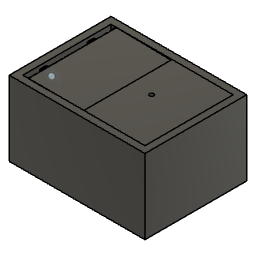
Useless box v2 (Autodesk Fusion 360 design; units mm, degrees)
Autodesk Fusion 360 part; units mm, degrees
sketch "Esquisse1" plane through (0, 0, 0) normal (0, 1, 0) x (1, 0, 0)
  line L0 (0, 0) -> (200, 0)
  line L1 (200, 0) -> (200, -150)
  line L2 (200, -150) -> (0, -150)
  line L3 (0, -150) -> (0, 0)
  line L4 (10, -10) -> (190, -10)
  line L5 (190, -10) -> (190, -140)
  line L6 (190, -140) -> (10, -140)
  line L7 (10, -140) -> (10, -10)
  dimension "d1" = 200
  dimension "d2" = 150
  constraint horizontal L0
  constraint vertical L1
  constraint horizontal L2
  constraint vertical L3
  constraint coincident L0.start L3.end
  constraint horizontal L4
  constraint vertical L5
  constraint horizontal L6
  constraint vertical L7
  measures "d1" distance of L0.start L0.end
  measures "d2" distance of L0 L2
sketch "Esquisse2" plane through (100, 0, 75) normal (0, 1, 0) x (1, 0, 0)
  line L0 (-90, 65) -> (90, 65)
  line L1 (90, 65) -> (90, -65)
  line L2 (90, -65) -> (-90, -65)
  line L3 (-90, -65) -> (-90, 65)
  constraint horizontal L0
  constraint vertical L1
  constraint horizontal L2
  constraint vertical L3
extrude "Extrusion1" add sketch "Esquisse1" along normal blind 20 contours L0 L1 L2 L3 | L4 L5 L6 L7 makes body 1
sketch "Esquisse3" plane through (100, 0, 75) normal (0, 1, 0) x (1, 0, 0)
extrude "Extrusion2" add sketch "Esquisse1" along normal blind 90 from surface at 20 bodies 1
sketch "Esquisse4" plane through (190, 0, 0) normal (-1, 0, 0) x (0, 0, 1)
  line L0 (10, 20) -> (140, 20)
  line L1 (140, 20) -> (140, 110)
  line L2 (140, 110) -> (10, 110)
  line L3 (10, 110) -> (10, 20)
  line L4 (10, 110) -> (140, 110)
  line L5 (140, 110) -> (140, 100)
  line L6 (140, 100) -> (10, 100)
  line L7 (10, 100) -> (10, 110)
  constraint horizontal L4
  constraint vertical L5
  constraint horizontal L6
  constraint vertical L7
  constraint coincident L1 L5.end
  constraint coincident L2.end L3.start
extrude "Extrusion3" add sketch "Esquisse4" along normal blind 90 separate body contours L1 L2 L3 L4 L5 L6 L7 makes body 2
sketch "Esquisse5" plane through (10, 0, 0) normal (1, 0, 0) x (0, 0, -1)
  line L0 (-140, 20) -> (-10, 20)
  line L1 (-10, 20) -> (-10, 110)
  line L2 (-10, 110) -> (-140, 110)
  line L3 (-140, 110) -> (-140, 20)
  line L4 (-115, 105) -> (-105, 105)
  line L5 (-105, 105) -> (-105, 90)
  line L6 (-105, 90) -> (-115, 90)
  line L7 (-115, 90) -> (-115, 105)
  line L8 (-35, 105) -> (-45, 105)
  line L9 (-45, 105) -> (-45, 90)
  line L10 (-45, 90) -> (-35, 90)
  line L11 (-35, 90) -> (-35, 105)
  constraint horizontal L4
  constraint vertical L5
  constraint horizontal L6
  constraint vertical L7
  constraint horizontal L8
  constraint vertical L9
  constraint horizontal L10
  constraint vertical L11
extrude "Extrusion4" add sketch "Esquisse5" along normal blind 20 separate body contours L4 L5 L6 L7 | L8 L9 L10 L11 makes body 3 at (16.6667, 100, 105) makes body 4 at (16.6667, 95, 35)
sketch "Esquisse6" plane through (0, 0, 105) normal (0, 0, -1) x (-1, 0, 0)
  line L0 (-10, 90) -> (-10, 105)
  line L1 (-10, 105) -> (-30, 105)
  line L2 (-30, 105) -> (-30, 90)
  line L3 (-30, 90) -> (-10, 90)
  circle A0 centre (-17.5, 95) radius 2.5
  dimension "d12" = 5
  measures "d12" diameter of A0
extrude "Extrusion5" cut sketch "Esquisse6" along normal blind 70 and the other way blind 10 contours A0 bodies 3 4
sketch "Esquisse7" plane through (0, 110, 0) normal (0, 1, 0) x (-1, 0, 0)
  line L0 (-190, 140) -> (-190, 10)
  line L1 (-190, 10) -> (-100, 10)
  line L2 (-100, 10) -> (-100, 140)
  line L3 (-100, 140) -> (-190, 140)
  circle A0 centre (-130, 70) radius 3
  dimension "d17" = 6
  measures "d17" diameter of A0
extrude "Extrusion6" cut sketch "Esquisse7" against normal blind 10 contours A0 bodies 2
sketch "Esquisse1 (2)" plane through (0, 110, 0) normal (0, 1, 0) x (-1, 0, 0) in component "couvercle"
  line L0 (-190, 140) -> (-10, 140)
  line L1 (-10, 140) -> (-10, 10)
  line L2 (-10, 10) -> (-190, 10)
  line L3 (-190, 10) -> (-190, 140)
  line L4 (0, 150) -> (-200, 150)
  line L5 (-200, 150) -> (-200, 0)
  line L6 (-200, 0) -> (0, 0)
  line L7 (0, 0) -> (0, 150)
  line L8 (-10, 114.9857) -> (-30, 114.9857)
  line L9 (-30, 114.9857) -> (-30, 105)
  line L10 (-30, 105) -> (-10, 105)
  line L11 (-10, 105) -> (-10, 114.9857)
  line L12 (-30, 35) -> (-10, 35)
  line L13 (-10, 35) -> (-10, 45)
  line L14 (-10, 45) -> (-30, 45)
  line L15 (-30, 45) -> (-30, 35)
  line L16 (-10, 103.8503) -> (-30, 103.8503)
  line L17 (-30, 103.8503) -> (-30, 46)
  line L18 (-30, 46) -> (-10, 46)
  line L19 (-10, 46) -> (-10, 103.8503)
  constraint horizontal L8
  constraint vertical L9
  constraint horizontal L10
  constraint vertical L11
  constraint coincident L1 L8.start
  constraint horizontal L12
  constraint vertical L13
  constraint horizontal L14
  constraint vertical L15
  constraint coincident L1 L13.end
  constraint horizontal L16
  constraint vertical L17
  constraint horizontal L18
  constraint vertical L19
  constraint coincident L1 L16.start
extrude "Extrusion7" cut 1 faces at (30, 100, 111.6667) along direction (-1, 0, 0) blind 6 on bodies 3 bodies 3
extrude "Extrusion8" cut 1 faces at (30, 100, 41.6667) along direction (-1, 0, 0) blind 6 on bodies 4 bodies 4
sketch "Esquisse8" plane through (0, 110, 0) normal (0, 1, 0) x (-1, 0, 0)
  line L0 (-10, 10) -> (-100, 10)
  line L1 (-100, 10) -> (-100, 140)
  line L2 (-100, 140) -> (-10, 140)
  line L3 (-10, 140) -> (-10, 10)
  constraint horizontal L0
  constraint vertical L1
  constraint horizontal L2
  constraint vertical L3
extrude "Extrusion1'" add sketch "Esquisse8" against normal blind 10 separate body makes body 5 in component "couvercle"
extrude "Extrusion2'" cut sketch "Esquisse1 (2)" against normal blind 5 from surface at -5 contours L1 L8 L9 L10 L11 bodies 5 in component "couvercle"
extrude "Extrusion3'" cut sketch "Esquisse1 (2)" against normal blind 5 from surface at -5 contours L1 L12 L13 L14 L15 bodies 5 in component "couvercle"
extrude "Extrusion4'" add sketch "Esquisse1 (2)" against normal blind 10 from surface at -10 contours L1 L16 L17 L18 L19 bodies 5 in component "couvercle"
fillet "Congé1" radius 8 tangency weight 0.25 1 edges at (10, 110, 75) on bodies 5 in component "couvercle"
chamfer "Chanfrein1" distance 3.5 distance2 10 1 edges at (100, 100, 75) measured on face at (76.6667, 100, 84.6168) on bodies 5 in component "couvercle"
sketch "Esquisse2 (2)" plane through (0, 0, 46) normal (0, 0, -1) x (-1, 0, 0) in component "couvercle"
  line L0 (-10, 100) -> (-30, 100)
  line L1 (-30, 100) -> (-30, 90)
  line L2 (-30, 90) -> (-10, 90)
  line L3 (-10, 90) -> (-10, 100)
  circle A0 centre (-17.5, 95) radius 2.5
extrude "Extrusion5'" cut sketch "Esquisse6" along normal blind 60 contours A0 bodies 5 in component "couvercle"
component "couvercle" placed x (0.766044, 0.642788, 0) y (-0.642788, 0.766044, 0) z (0, 0, 1) at (65.159, 10.977, 0.1497)
